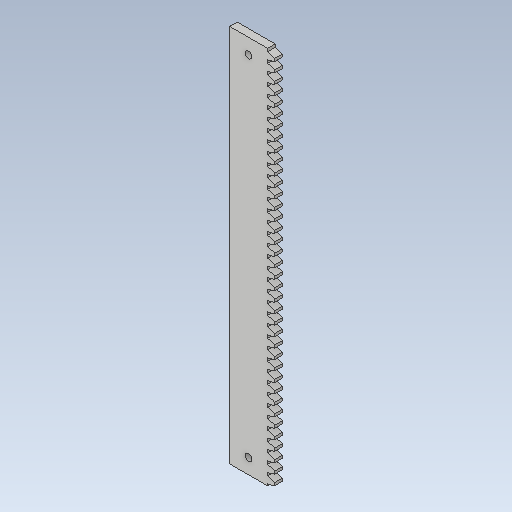
# Autodesk Inventor part: Rack
Saved by Autodesk Inventor 2020.1 (Build 241239000, 239)
## iProperties
Created: 2019-10-24
Part Number: Rack
Material: Generic
Document SubType Name: Modeling
Designer: ajtan
Density: 1 g/cm^3
Appearance: Default
Author: ajtan
Autodesk Inventor part; units mm, degrees
ref_plane "YZ Plane" through (0, 0, 0) normal (1, 0, 0) x (0, 1, 0)
ref_plane "XZ Plane" through (0, 0, 0) normal (0, 1, 0) x (-1, 0, 0)
ref_plane "XY Plane" through (0, 0, 0) normal (0, 0, 1) x (1, 0, 0)
sketch "Sketch1" plane through (0, 0, 0) normal (0, 0, 1) x (1, 0, 0)
  line L0 (0, 0) -> (25.4, 0)
  line L1 (25.4, 254) -> (0, 254)
  line L2 (0, 254) -> (0, 0)
  arc A0 (25.4, 247.3659) -> (30.2405, 248.7636) centre (21.987, 268.2656) ccw
  arc A1 (30.2403, 250.5461) -> (25.3995, 251.942) centre (21.9941, 231.0411) ccw
  line L3 (25.3995, 251.942) -> (25.3995, 254)
  line L4 (12.7, 261.3016) -> (12.7, -25.6207) construction
  circle A2 centre (12.7, 243.84) radius 2.286
  line L5 (0, 127) -> (12.7, 127) construction
  circle A3 centre (12.7, 10.16) radius 2.286
  line L6 (30.2403, 250.5461) -> (30.2405, 248.7636)
  arc A4 (30.2403, 243.8913) -> (25.3995, 245.2872) centre (21.9941, 224.3863) ccw
  line L7 (30.2403, 243.8913) -> (30.2405, 242.1088)
  arc A5 (25.4, 240.7111) -> (30.2405, 242.1088) centre (21.987, 261.6108) ccw
  arc A6 (30.2403, 237.2365) -> (25.3995, 238.6324) centre (21.9941, 217.7315) ccw
  line L8 (30.2403, 237.2365) -> (30.2405, 235.454)
  arc A7 (25.4, 234.0563) -> (30.2405, 235.454) centre (21.987, 254.956) ccw
  arc A8 (30.2403, 230.5817) -> (25.3995, 231.9776) centre (21.9941, 211.0767) ccw
  line L9 (30.2403, 230.5817) -> (30.2405, 228.7992)
  arc A9 (25.4, 227.4015) -> (30.2405, 228.7992) centre (21.987, 248.3012) ccw
  arc A10 (30.2403, 223.9269) -> (25.3995, 225.3228) centre (21.9941, 204.4219) ccw
  line L10 (30.2403, 223.9269) -> (30.2405, 222.1444)
  arc A11 (25.4, 220.7467) -> (30.2405, 222.1444) centre (21.987, 241.6464) ccw
  arc A12 (30.2403, 217.2721) -> (25.3995, 218.668) centre (21.9941, 197.7671) ccw
  line L11 (30.2403, 217.2721) -> (30.2405, 215.4896)
  arc A13 (25.4, 214.0919) -> (30.2405, 215.4896) centre (21.987, 234.9916) ccw
  arc A14 (30.2403, 210.6173) -> (25.3995, 212.0132) centre (21.9941, 191.1123) ccw
  line L12 (30.2403, 210.6173) -> (30.2405, 208.8348)
  arc A15 (25.4, 207.4371) -> (30.2405, 208.8348) centre (21.987, 228.3368) ccw
  arc A16 (30.2403, 203.9625) -> (25.3995, 205.3584) centre (21.9941, 184.4575) ccw
  line L13 (30.2403, 203.9625) -> (30.2405, 202.18)
  arc A17 (25.4, 200.7823) -> (30.2405, 202.18) centre (21.987, 221.682) ccw
  arc A18 (30.2403, 197.3077) -> (25.3995, 198.7036) centre (21.9941, 177.8027) ccw
  line L14 (30.2403, 197.3077) -> (30.2405, 195.5252)
  arc A19 (25.4, 194.1275) -> (30.2405, 195.5252) centre (21.987, 215.0272) ccw
  arc A20 (30.2403, 190.6529) -> (25.3995, 192.0488) centre (21.9941, 171.1479) ccw
  line L15 (30.2403, 190.6529) -> (30.2405, 188.8704)
  arc A21 (25.4, 187.4727) -> (30.2405, 188.8704) centre (21.987, 208.3724) ccw
  arc A22 (30.2403, 183.9981) -> (25.3995, 185.394) centre (21.9941, 164.4931) ccw
  line L16 (30.2403, 183.9981) -> (30.2405, 182.2156)
  arc A23 (25.4, 180.8179) -> (30.2405, 182.2156) centre (21.987, 201.7176) ccw
  arc A24 (30.2403, 177.3433) -> (25.3995, 178.7392) centre (21.9941, 157.8383) ccw
  line L17 (30.2403, 177.3433) -> (30.2405, 175.5608)
  arc A25 (25.4, 174.1631) -> (30.2405, 175.5608) centre (21.987, 195.0628) ccw
  arc A26 (30.2403, 170.6885) -> (25.3995, 172.0844) centre (21.9941, 151.1835) ccw
  line L18 (30.2403, 170.6885) -> (30.2405, 168.906)
  arc A27 (25.4, 167.5083) -> (30.2405, 168.906) centre (21.987, 188.408) ccw
  arc A28 (30.2403, 164.0337) -> (25.3995, 165.4296) centre (21.9941, 144.5287) ccw
  line L19 (30.2403, 164.0337) -> (30.2405, 162.2512)
  arc A29 (25.4, 160.8535) -> (30.2405, 162.2512) centre (21.987, 181.7532) ccw
  arc A30 (30.2403, 157.3789) -> (25.3995, 158.7748) centre (21.9941, 137.8739) ccw
  line L20 (30.2403, 157.3789) -> (30.2405, 155.5964)
  arc A31 (25.4, 154.1987) -> (30.2405, 155.5964) centre (21.987, 175.0984) ccw
  arc A32 (30.2403, 150.7241) -> (25.3995, 152.12) centre (21.9941, 131.2191) ccw
  line L21 (30.2403, 150.7241) -> (30.2405, 148.9416)
  arc A33 (25.4, 147.5439) -> (30.2405, 148.9416) centre (21.987, 168.4436) ccw
  arc A34 (30.2403, 144.0693) -> (25.3995, 145.4652) centre (21.9941, 124.5643) ccw
  line L22 (30.2403, 144.0693) -> (30.2405, 142.2868)
  arc A35 (25.4, 140.8891) -> (30.2405, 142.2868) centre (21.987, 161.7888) ccw
  arc A36 (30.2403, 137.4145) -> (25.3995, 138.8104) centre (21.9941, 117.9095) ccw
  line L23 (30.2403, 137.4145) -> (30.2405, 135.632)
  arc A37 (25.4, 134.2343) -> (30.2405, 135.632) centre (21.987, 155.134) ccw
  arc A38 (30.2403, 130.7597) -> (25.3995, 132.1556) centre (21.9941, 111.2547) ccw
  line L24 (30.2403, 130.7597) -> (30.2405, 128.9772)
  arc A39 (25.4, 127.5795) -> (30.2405, 128.9772) centre (21.987, 148.4792) ccw
  arc A40 (30.2403, 124.1049) -> (25.3995, 125.5008) centre (21.9941, 104.5999) ccw
  line L25 (30.2403, 124.1049) -> (30.2405, 122.3224)
  arc A41 (25.4, 120.9247) -> (30.2405, 122.3224) centre (21.987, 141.8244) ccw
  arc A42 (30.2403, 117.4501) -> (25.3995, 118.846) centre (21.9941, 97.9451) ccw
  line L26 (30.2403, 117.4501) -> (30.2405, 115.6676)
  arc A43 (25.4, 114.2699) -> (30.2405, 115.6676) centre (21.987, 135.1696) ccw
  arc A44 (30.2403, 110.7953) -> (25.3995, 112.1912) centre (21.9941, 91.2903) ccw
  line L27 (30.2403, 110.7953) -> (30.2405, 109.0128)
  arc A45 (25.4, 107.6151) -> (30.2405, 109.0128) centre (21.987, 128.5148) ccw
  arc A46 (30.2403, 104.1405) -> (25.3995, 105.5364) centre (21.9941, 84.6355) ccw
  line L28 (30.2403, 104.1405) -> (30.2405, 102.358)
  arc A47 (25.4, 100.9603) -> (30.2405, 102.358) centre (21.987, 121.86) ccw
  arc A48 (30.2403, 97.4857) -> (25.3995, 98.8816) centre (21.9941, 77.9807) ccw
  line L29 (30.2403, 97.4857) -> (30.2405, 95.7032)
  arc A49 (25.4, 94.3055) -> (30.2405, 95.7032) centre (21.987, 115.2052) ccw
  arc A50 (30.2403, 90.8309) -> (25.3995, 92.2268) centre (21.9941, 71.3259) ccw
  line L30 (30.2403, 90.8309) -> (30.2405, 89.0484)
  arc A51 (25.4, 87.6507) -> (30.2405, 89.0484) centre (21.987, 108.5504) ccw
  arc A52 (30.2403, 84.1761) -> (25.3995, 85.572) centre (21.9941, 64.6711) ccw
  line L31 (30.2403, 84.1761) -> (30.2405, 82.3936)
  arc A53 (25.4, 80.9959) -> (30.2405, 82.3936) centre (21.987, 101.8956) ccw
  arc A54 (30.2403, 77.5213) -> (25.3995, 78.9172) centre (21.9941, 58.0163) ccw
  line L32 (30.2403, 77.5213) -> (30.2405, 75.7388)
  arc A55 (25.4, 74.3411) -> (30.2405, 75.7388) centre (21.987, 95.2408) ccw
  arc A56 (30.2403, 70.8665) -> (25.3995, 72.2624) centre (21.9941, 51.3615) ccw
  line L33 (30.2403, 70.8665) -> (30.2405, 69.084)
  arc A57 (25.4, 67.6863) -> (30.2405, 69.084) centre (21.987, 88.586) ccw
  arc A58 (30.2403, 64.2117) -> (25.3995, 65.6076) centre (21.9941, 44.7067) ccw
  line L34 (30.2403, 64.2117) -> (30.2405, 62.4292)
  arc A59 (25.4, 61.0315) -> (30.2405, 62.4292) centre (21.987, 81.9312) ccw
  arc A60 (30.2403, 57.5569) -> (25.3995, 58.9528) centre (21.9941, 38.0519) ccw
  line L35 (30.2403, 57.5569) -> (30.2405, 55.7744)
  arc A61 (25.4, 54.3767) -> (30.2405, 55.7744) centre (21.987, 75.2764) ccw
  arc A62 (30.2403, 50.9021) -> (25.3995, 52.298) centre (21.9941, 31.3971) ccw
  line L36 (30.2403, 50.9021) -> (30.2405, 49.1196)
  arc A63 (25.4, 47.7219) -> (30.2405, 49.1196) centre (21.987, 68.6216) ccw
  arc A64 (30.2403, 44.2473) -> (25.3995, 45.6432) centre (21.9941, 24.7423) ccw
  line L37 (30.2403, 44.2473) -> (30.2405, 42.4648)
  arc A65 (25.4, 41.0671) -> (30.2405, 42.4648) centre (21.987, 61.9668) ccw
  arc A66 (30.2403, 37.5925) -> (25.3995, 38.9884) centre (21.9941, 18.0875) ccw
  line L38 (30.2403, 37.5925) -> (30.2405, 35.81)
  arc A67 (25.4, 34.4123) -> (30.2405, 35.81) centre (21.987, 55.312) ccw
  arc A68 (30.2403, 30.9377) -> (25.3995, 32.3336) centre (21.9941, 11.4327) ccw
  line L39 (30.2403, 30.9377) -> (30.2405, 29.1552)
  arc A69 (25.4, 27.7575) -> (30.2405, 29.1552) centre (21.987, 48.6572) ccw
  arc A70 (30.2403, 24.2829) -> (25.3995, 25.6788) centre (21.9941, 4.7779) ccw
  line L40 (30.2403, 24.2829) -> (30.2405, 22.5004)
  arc A71 (25.4, 21.1027) -> (30.2405, 22.5004) centre (21.987, 42.0024) ccw
  arc A72 (30.2403, 17.6281) -> (25.3995, 19.024) centre (21.9941, -1.8769) ccw
  line L41 (30.2403, 17.6281) -> (30.2405, 15.8456)
  arc A73 (25.4, 14.4479) -> (30.2405, 15.8456) centre (21.987, 35.3476) ccw
  arc A74 (30.2403, 10.9733) -> (25.3995, 12.3692) centre (21.9941, -8.5317) ccw
  line L42 (30.2403, 10.9733) -> (30.2405, 9.1908)
  arc A75 (25.4, 7.7931) -> (30.2405, 9.1908) centre (21.987, 28.6928) ccw
  arc A76 (30.2403, 4.3185) -> (25.3995, 5.7144) centre (21.9941, -15.1865) ccw
  line L43 (30.2403, 4.3185) -> (30.2405, 2.536)
  arc A77 (25.4, 1.1383) -> (30.2405, 2.536) centre (21.987, 22.038) ccw
  line L44 (25.4, 247.3659) -> (25.4, 245.2871)
  line L45 (25.4, 240.7111) -> (25.4, 238.6323)
  line L46 (25.4, 234.0563) -> (25.4, 231.9775)
  line L47 (25.4, 227.4015) -> (25.4, 225.3227)
  line L48 (25.4, 220.7467) -> (25.4, 218.6679)
  line L49 (25.4, 214.0919) -> (25.4, 212.0131)
  line L50 (25.4, 207.4371) -> (25.4, 205.3583)
  line L51 (25.4, 200.7823) -> (25.4, 198.7035)
  line L52 (25.4, 194.1275) -> (25.4, 192.0487)
  line L53 (25.4, 187.4727) -> (25.4, 185.3939)
  line L54 (25.4, 180.8179) -> (25.4, 178.7391)
  line L55 (25.4, 174.1631) -> (25.4, 172.0843)
  line L56 (25.4, 167.5083) -> (25.4, 165.4295)
  line L57 (25.4, 160.8535) -> (25.4, 158.7747)
  line L58 (25.4, 154.1987) -> (25.4, 152.1199)
  line L59 (25.4, 147.5439) -> (25.4, 145.4651)
  line L60 (25.4, 140.8891) -> (25.4, 138.8103)
  line L61 (25.4, 134.2343) -> (25.4, 132.1555)
  line L62 (25.4, 127.5795) -> (25.4, 125.5007)
  line L63 (25.4, 120.9247) -> (25.4, 118.8459)
  line L64 (25.4, 114.2699) -> (25.4, 112.1911)
  line L65 (25.4, 107.6151) -> (25.4, 105.5363)
  line L66 (25.4, 100.9603) -> (25.4, 98.8815)
  line L67 (25.4, 94.3055) -> (25.4, 92.2267)
  line L68 (25.4, 87.6507) -> (25.4, 85.5719)
  line L69 (25.4, 80.9959) -> (25.4, 78.9171)
  line L70 (25.4, 74.3411) -> (25.4, 72.2623)
  line L71 (25.4, 67.6863) -> (25.4, 65.6075)
  line L72 (25.4, 61.0315) -> (25.4, 58.9527)
  line L73 (25.4, 54.3767) -> (25.4, 52.2979)
  line L74 (25.4, 47.7219) -> (25.4, 45.6431)
  line L75 (25.4, 41.0671) -> (25.4, 38.9883)
  line L76 (25.4, 34.4123) -> (25.4, 32.3335)
  line L77 (25.4, 27.7575) -> (25.4, 25.6787)
  line L78 (25.4, 21.1027) -> (25.4, 19.0239)
  line L79 (25.4, 14.4479) -> (25.4, 12.3691)
  line L80 (25.4, 7.7931) -> (25.4, 5.7143)
  line L81 (25.4, 1.1383) -> (25.4, 0)
  dimension "d0" = 25.4
  dimension "d25" = 12.7
  dimension "d26" = 4.572
  dimension "d27" = 10.16
  dimension "d28" = 127
  dimension "d38" = 254
  dimension "d48" = 25.3995
  dimension "d51" = 6.6548
  constraints: 189 point on circle, 164 end point, 78 centre point, 39 vertical, 3 parallel, 3 point on line, 1 horizontal, 1 midpoint, 1 perpendicular, 1 symmetric about line, 334 other
  measures "d0" distance of L1.end L1.start
  measures "d25" distance between parallel lines of L2 L4
  measures "d26" diameter of A2
  measures "d27" distance from line of L1 A2.centre
  measures "d28" distance between parallel lines of L0 L5
  measures "d38" distance between parallel lines of L1 L0
  measures "d48" distance between parallel lines of L2 L3
  measures "d51" distance of L6.start L7.start
extrude "Extrusion3" add sketch "Sketch1" along normal blind 5.08
body "Solid3"
